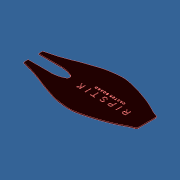
# Autodesk Inventor part: Front Board Cover
Saved by Autodesk Inventor 2018 (Build 220112000, 112)
## iProperties
Created: 2018-03-02
Part Number: Front Board Cover
Material: Generic
Document SubType Name: Modeling
Designer: 232963
Density: 1 g/cm^3
Appearance: Default
Author: 232963
Autodesk Inventor part; units mm, degrees
ref_plane "YZ Plane" through (0, 0, 0) normal (1, 0, 0) x (0, 1, 0)
ref_plane "XZ Plane" through (0, 0, 0) normal (0, 1, 0) x (-1, 0, 0)
ref_plane "XY Plane" through (0, 0, 0) normal (0, 0, 1) x (1, 0, 0)
sketch "Sketch1" plane through (0, 0, 0) normal (0, 0, 1) x (1, 0, 0)
  line L0 (-34.346, 0) -> (308.554, 0)
  line L1 (-34.346, 2.794) -> (-34.346, 0)
  line L2 (-34.346, 2.794) -> (308.554, 2.794)
  line L3 (308.554, 2.794) -> (308.554, 0)
  point P0 (0, 0)
  dimension "d102" = 342.9
  constraints: 8 end point, 1 horizontal, 1 vertical, 1 other
  measures "d102" distance from line of L0.end L1
extrude "Extrusion1" add sketch "Sketch1" along normal blind 161.925
sketch "Sketch2" plane through (-34.346, 2.794, 0) normal (0, 1, 0) x (1, 0, 0)
  line L0 (0, 0) -> (0, -161.925) projected
  line L1 (0, -80.9625) -> (355.6, -80.9625)
  line L2 (342.9, 0) -> (0, 0) projected
  line L3 (0, 0) -> (342.9, 0) projected
  spline S0 degree 4 poles (190.5, 0) (176.6775, 0) (146.1194, -4.9047) (146.8521, -3.1203) (83.6356, -24.6252) (79.4605, -26.74) (68.0118, -31.1235) (63.3839, -33.2828) (38.0924, -42.0424) (22.0487, -47.0453) (18.7736, -46.718) (0.7177, -52.7069) (0, -52.4002) knots 0 0 0 0 0 0.204521 0.323697 0.422378 0.506708 0.581474 0.662125 0.742434 0.828574 1 1 1 1 1
  line L4 (0, -52.4002) -> (0, 0)
  line L5 (190.5, 0) -> (0, 0)
  line L6 (342.9, 0) -> (342.9, -161.925) projected
  spline S1 degree 4 poles (190.5, 0) (208.4411, 0) (251.3479, -12.7353) (261.4383, -16.5213) (279.9875, -22.867) (307.7965, -33.882) (329.1012, -47.2629) (336.8853, -48.836) (342.9, -49.53) knots 0 0 0 0 0 0.297202 0.471636 0.622976 0.773941 1 1 1 1 1
  line L7 (324.9507, -47.459) -> (360.8493, -51.601) construction
  arc A0 (328.7385, -47.0401) -> (357.2564, -50.3305) centre (356.8343, 71.2391) ccw construction
  line L8 (199.9843, 0) -> (190.5, 0)
  point P0 (34.346, 0)
  point P1 (0, -112.0775)
  point P2 (184.15, -161.925)
  point P3 (6.35, -50.8)
  point P4 (19.05, -47.244)
  point P5 (25.4, -45.72)
  point P6 (63.5, -33.02)
  point P7 (38.1, -41.91)
  point P8 (76.2, -27.94)
  point P9 (127, -10.16)
  point P10 (152.4, -3.81)
  point P11 (69.85, -30.48)
  point P12 (82.55, -25.4)
  point P13 (266.7, -18.288)
  point P14 (279.4, -22.86)
  point P15 (304.8, -33.655)
  point P16 (330.2, -46.355)
  point P17 (342.9, -49.53)
  dimension "d8" = 31.115
  dimension "d9" = 184.15
  dimension "d12" = 52.4002
  dimension "d13" = 50.8
  dimension "d15" = 47.244
  dimension "d16" = 6.35
  dimension "d19" = 6.35
  dimension "d20" = 45.72
  dimension "d31" = 41.91
  dimension "d35" = 33.02
  dimension "d37" = 27.94
  dimension "d38" = 12.7
  dimension "d45" = 10.16
  dimension "d49" = 3.81
  dimension "d57" = 30.48
  dimension "d58" = 6.35
  dimension "d60" = 25.4
  dimension "d89" = 190.5
  dimension "d95" = 12.7
  dimension "d96" = 12.7
  dimension "d107" = 13.97
  dimension "d108" = 18.288
  dimension "d109" = 22.86
  dimension "d111" = 33.655
  dimension "d112" = 46.355
  dimension "d113" = 25.4
  dimension "d114" = 49.53
  constraints: 10 end point, 5 point on line, 3 collinear, 3 midpoint, 2 horizontal, 1 centre point, 1 point on circle, 21 other
  measures "d8" distance of point (0, -112.078) L1.start
  measures "d9" distance of L0.end point (184.15, -161.925)
  measures "d12" distance from line of L2 L4.start
  measures "d13" distance from line of L2 point (6.35, -50.8)
  measures "d15" distance from line of L2 point (19.05, -47.244)
  measures "d16" horizontal distance of point (6.35, -50.8) L4.start
  measures "d19" horizontal distance of point (25.4, -45.72) point (19.05, -47.244)
  measures "d20" distance from line of L2 point (25.4, -45.72)
  measures "d31" distance from line of L2 point (38.1, -41.91)
  measures "d35" distance from line of L2 point (63.5, -33.02)
  measures "d37" distance from line of L2 point (76.2, -27.94)
  measures "d38" horizontal distance of point (63.5, -33.02) point (76.2, -27.94)
  measures "d45" distance from line of L2 point (127, -10.16)
  measures "d49" distance from line of L2 point (152.4, -3.81)
  measures "d57" distance from line of L2 point (69.85, -30.48)
  measures "d58" horizontal distance of point (76.2, -27.94) point (69.85, -30.48)
  measures "d60" distance from line of L2 point (82.55, -25.4)
  measures "d89" horizontal distance of L5.start L4.start
  measures "d95" horizontal distance of point (266.7, -18.288) point (254, -13.97)
  measures "d96" horizontal distance of point (279.4, -22.86) point (266.7, -18.288)
  measures "d107" distance from line of L2 point (254, -13.97)
  measures "d108" distance from line of L2 point (266.7, -18.288)
  measures "d109" distance from line of L2 point (279.4, -22.86)
  measures "d111" distance from line of L2 point (304.8, -33.655)
  measures "d112" distance from line of L2 point (330.2, -46.355)
  measures "d113" horizontal distance of point (304.8, -33.655) point (330.2, -46.355)
  measures "d114" distance from line of point (342.9, -49.53) L2
extrude "Extrusion2" cut sketch "Sketch2" against normal blind 25.4 contours L2 S0 L0 | L2 L6 S1
ref_plane "Work Plane2" through (0, 0, 80.9625) normal (0, 0, -1) x (-1, 0, 0)
mirror "Mirror1" about plane through (0, 0, 80.9625) normal (0, 0, -1) of "Extrusion2"
sketch "Sketch3" plane through (308.554, 2.794, 161.925) normal (0, 1, 0) x (1, 0, 0)
  line L0 (-342.9, 109.5248) -> (-342.9, 52.4002) projected
  line L1 (-342.9, 97.6249) -> (-273.05, 97.6249)
  line L2 (-234.95, 96.0374) -> (-234.95, 9.9368) construction
  line L3 (-273.05, 65.8749) -> (-342.9, 65.8749)
  line L4 (-342.9, 65.8749) -> (-342.9, 97.6249)
  line L5 (-273.05, 97.6249) -> (-273.05, 65.8749)
  arc A0 (-273.05, 65.8749) -> (-238.76, 74.1299) centre (-273.05, 141.2201) ccw
  arc A1 (-238.76, 89.3699) -> (-273.05, 97.6249) centre (-273.05, 22.2797) ccw
  line L6 (-238.76, 96.0374) -> (-238.76, 64.2874) construction
  spline S0 degree 4 poles (-238.76, 74.1299) (-236.6016, 75.2331) (-232.3793, 77.6246) (-232.3793, 85.8752) (-236.6016, 88.2667) (-238.76, 89.3699) knots 0 0 0 0 0 0.5 1 1 1 1 1
  point P0 (-308.554, 161.925)
  dimension "d75" = 31.75
  dimension "d78" = 57.1246
  dimension "d79" = 11.8999
  dimension "d80" = 38.1
  dimension "d81" = 15.24
  dimension "d82" = 0
  dimension "d83" = 8.255
  dimension "d84" = 3.81
  dimension "d85" = 0
  dimension "d86" = 107.95
  constraints: 12 end point, 4 point on circle, 2 centre point, 2 parallel, 2 perpendicular, 2 tangent, 1 horizontal, 1 point on line, 1 vertical, 4 other
  measures "d75" distance between parallel lines of L3 L1
  measures "d78" distance of L0.end L0.start
  measures "d79" distance of L0.start L1.start
  measures "d80" distance between parallel lines of L2 L5
  measures "d81" distance of A0.end A1.start
  measures "d82" horizontal distance of A0.end A1.start
  measures "d83" distance from line of A0.end L3
  measures "d84" distance between parallel lines of L6 L2
  measures "d85" distance from line of L6 A1.start
  measures "d86" distance from line of L2 L3.end
extrude "Extrusion3" cut sketch "Sketch3" against normal blind 25.4
fillet "Fillet1" radius 5.715 1 edges at (308.554, 1.397, 49.53)
fillet "Fillet2" radius 5.715 1 edges at (308.554, 1.397, 112.395)
sketch "Sketch4" plane through (-34.346, 2.794, 64.3001) normal (0, 1, 0) x (1, 0, 0)
  line L0 (292.9191, -30.9357) -> (86.9557, -30.9357) construction
  line L1 (86.9557, -30.9357) -> (86.9557, -10.5653) construction
  line L2 (86.9557, -10.5653) -> (292.9191, -10.5653) construction
  line L3 (292.9191, -10.5653) -> (292.9191, -30.9357) construction
  line L4 (261.7969, -5.5259) -> (138.9964, -5.5259) construction
  line L5 (138.9964, -5.5259) -> (138.9964, 7.7104) construction
  line L6 (138.9964, 7.7104) -> (261.7969, 7.7104) construction
  line L7 (261.7969, 7.7104) -> (261.7969, -5.5259) construction
  spline S0 degree 2 poles (279.0348, -25.5302) (279.0348, -22.9286) (280.7333, -21.6346) knots 0 0 0 1 1 1
  spline S1 degree 2 poles (280.7333, -21.6346) (281.9061, -20.7584) (283.0114, -20.7584) knots 0 0 0 1 1 1
  line L8 (283.0114, -20.7584) -> (283.9146, -20.7584)
  line L9 (283.9146, -20.7584) -> (279.1831, -14.0993)
  spline S2 degree 2 poles (279.1831, -14.0993) (279.0348, -13.8701) (279.0348, -13.614) knots 0 0 0 1 1 1
  spline S3 degree 2 poles (279.0348, -13.614) (279.0348, -13.304) (279.5201, -12.8187) (279.8301, -12.8187) knots 0 0 0 1 2 2 2
  spline S4 degree 2 poles (279.8301, -12.8187) (280.2211, -12.8187) (280.4502, -13.1557) knots 0 0 0 1 1 1
  line L10 (280.4502, -13.1557) -> (285.8961, -20.7584)
  line L11 (285.8961, -20.7584) -> (289.9131, -20.7584)
  line L12 (289.9131, -20.7584) -> (289.9131, -13.641)
  spline S5 degree 2 poles (289.9131, -13.641) (289.9131, -12.8187) (290.7084, -12.8187) knots 0 0 0 1 1 1
  spline S6 degree 2 poles (290.7084, -12.8187) (291.5172, -12.8187) (291.5172, -13.641) knots 0 0 0 1 1 1
  line L13 (291.5172, -13.641) -> (291.5172, -30.4909)
  line L14 (291.5172, -30.4909) -> (283.982, -30.4909)
  spline S7 degree 2 poles (283.982, -30.4909) (281.9735, -30.4909) (280.5581, -29.1968) knots 0 0 0 1 1 1
  spline S8 degree 2 poles (280.5581, -29.1968) (279.0348, -27.8084) (279.0348, -25.5302) knots 0 0 0 1 1 1
  spline S9 degree 2 poles (280.612, -25.5302) (280.612, -27.0804) (281.6365, -28.0375) knots 0 0 0 1 1 1
  spline S10 degree 2 poles (281.6365, -28.0375) (282.5935, -28.8867) (283.982, -28.8867) knots 0 0 0 1 1 1
  line L15 (283.982, -28.8867) -> (289.9131, -28.8867)
  line L16 (289.9131, -28.8867) -> (289.9131, -22.3894)
  line L17 (289.9131, -22.3894) -> (283.0114, -22.3894)
  spline S11 degree 2 poles (283.0114, -22.3894) (282.3374, -22.3894) (281.623, -23.0095) knots 0 0 0 1 1 1
  spline S12 degree 2 poles (281.623, -23.0095) (280.612, -23.8587) (280.612, -25.5302) knots 0 0 0 1 1 1
  spline S13 degree 2 poles (263.0881, -13.641) (263.0881, -12.8187) (263.8699, -12.8187) knots 0 0 0 1 1 1
  spline S14 degree 2 poles (263.8699, -12.8187) (264.6653, -12.8187) (264.6653, -13.641) knots 0 0 0 1 1 1
  line L18 (264.6653, -13.641) -> (264.6653, -29.7225)
  spline S15 degree 2 poles (264.6653, -29.7225) (264.6653, -30.5448) (263.8699, -30.5448) knots 0 0 0 1 1 1
  spline S16 degree 2 poles (263.8699, -30.5448) (263.0881, -30.5448) (263.0881, -29.7225) knots 0 0 0 1 1 1
  line L19 (263.0881, -29.7225) -> (263.0881, -13.641)
  spline S17 degree 2 poles (236.6944, -25.9481) (236.6944, -23.9801) (237.7324, -22.8208) knots 0 0 0 1 1 1
  spline S18 degree 2 poles (237.7324, -22.8208) (238.8108, -21.5806) (240.7519, -21.5806) knots 0 0 0 1 1 1
  line L20 (240.7519, -21.5806) -> (246.373, -21.5806)
  line L21 (246.373, -21.5806) -> (246.373, -13.614)
  spline S19 degree 2 poles (246.373, -13.614) (246.373, -12.7917) (247.1548, -12.7917) knots 0 0 0 1 1 1
  spline S20 degree 2 poles (247.1548, -12.7917) (247.9502, -12.7917) (247.9502, -13.614) knots 0 0 0 1 1 1
  line L22 (247.9502, -13.614) -> (247.9502, -30.5178)
  line L23 (247.9502, -30.5178) -> (241.1832, -30.5178)
  spline S21 degree 2 poles (241.1832, -30.5178) (238.9186, -30.5178) (237.7594, -29.2237) knots 0 0 0 1 1 1
  spline S22 degree 2 poles (237.7594, -29.2237) (236.6944, -28.0375) (236.6944, -25.9481) knots 0 0 0 1 1 1
  spline S23 degree 2 poles (238.2716, -25.9481) (238.2716, -28.9137) (241.1832, -28.9137) knots 0 0 0 1 1 1
  line L24 (241.1832, -28.9137) -> (246.373, -28.9137)
  line L25 (246.373, -28.9137) -> (246.373, -23.2117)
  line L26 (246.373, -23.2117) -> (240.7519, -23.2117)
  spline S24 degree 2 poles (240.7519, -23.2117) (239.5657, -23.2117) (238.2716, -24.708) (238.2716, -25.9481) knots 0 0 0 1 2 2 2
  spline S25 degree 2 poles (211.7836, -17.5367) (211.7836, -12.6839) (217.9978, -12.6839) knots 0 0 0 1 1 1
  spline S26 degree 2 poles (217.9978, -12.6839) (221.7452, -12.6839) (223.7807, -16.4043) knots 0 0 0 1 1 1
  spline S27 degree 2 poles (223.7807, -16.4043) (223.8885, -16.6065) (223.8885, -16.8357) knots 0 0 0 1 1 1
  spline S28 degree 2 poles (223.8885, -16.8357) (223.8885, -17.1997) (223.4032, -17.7389) (223.0932, -17.7389) knots 0 0 0 1 2 2 2
  spline S29 degree 2 poles (223.0932, -17.7389) (222.7293, -17.7389) (222.5271, -17.3345) knots 0 0 0 1 1 1
  spline S30 degree 2 poles (222.5271, -17.3345) (221.8531, -15.9056) (219.3728, -14.288) (218.0113, -14.288) knots 0 0 0 1 2 2 2
  spline S31 degree 2 poles (218.0113, -14.288) (213.3877, -14.288) (213.3877, -17.5097) knots 0 0 0 1 1 1
  spline S32 degree 2 poles (213.3877, -17.5097) (213.3877, -18.8577) (214.7222, -19.7608) knots 0 0 0 1 1 1
  spline S33 degree 2 poles (214.7222, -19.7608) (215.6119, -20.3809) (217.7956, -21.1493) knots 0 0 0 1 1 1
  spline S34 degree 2 poles (217.7956, -21.1493) (220.7881, -22.2142) (221.8261, -22.9286) knots 0 0 0 1 1 1
  spline S35 degree 2 poles (221.8261, -22.9286) (223.7537, -24.2497) (223.7537, -26.366) knots 0 0 0 1 1 1
  spline S36 degree 2 poles (223.7537, -26.366) (223.7537, -28.6576) (222.0283, -29.8169) knots 0 0 0 1 1 1
  spline S37 degree 2 poles (222.0283, -29.8169) (220.6399, -30.7739) (218.3618, -30.8548) knots 0 0 0 1 1 1
  spline S38 degree 2 poles (218.3618, -30.8548) (216.2724, -30.9357) (214.7222, -30.0325) knots 0 0 0 1 1 1
  spline S39 degree 2 poles (214.7222, -30.0325) (213.0507, -29.0485) (212.4845, -27.1883) knots 0 0 0 1 1 1
  spline S40 degree 2 poles (212.4845, -27.1883) (212.4306, -27.0535) (212.4306, -26.9322) knots 0 0 0 1 1 1
  spline S41 degree 2 poles (212.4306, -26.9322) (212.4306, -26.2042) (213.2529, -26.2042) knots 0 0 0 1 1 1
  spline S42 degree 2 poles (213.2529, -26.2042) (213.846, -26.2042) (214.0347, -26.7704) knots 0 0 0 1 1 1
  spline S43 degree 2 poles (214.0347, -26.7704) (214.4121, -27.9566) (216.8385, -29.3046) (218.3078, -29.2507) knots 0 0 0 1 2 2 2
  spline S44 degree 2 poles (218.3078, -29.2507) (222.1766, -29.1024) (222.1766, -26.4064) knots 0 0 0 1 1 1
  spline S45 degree 2 poles (222.1766, -26.4064) (222.1766, -24.6271) (219.4941, -23.4948) knots 0 0 0 1 1 1
  spline S46 degree 2 poles (219.4941, -23.4948) (216.9868, -22.5107) (214.4661, -21.5402) knots 0 0 0 1 1 1
  spline S47 degree 2 poles (214.4661, -21.5402) (211.7836, -20.0709) (211.7836, -17.5367) knots 0 0 0 1 1 1
  line L27 (186.5492, -28.8463) -> (191.5233, -28.8463)
  line L28 (191.5233, -28.8463) -> (191.5233, -13.1961)
  spline S48 degree 2 poles (191.5233, -13.1961) (191.5233, -12.3739) (192.3455, -12.3739) knots 0 0 0 1 1 1
  spline S49 degree 2 poles (192.3455, -12.3739) (193.1813, -12.3739) (193.1813, -13.1961) knots 0 0 0 1 1 1
  line L29 (193.1813, -13.1961) -> (193.1813, -28.8463)
  line L30 (193.1813, -28.8463) -> (198.1689, -28.8463)
  spline S50 degree 2 poles (198.1689, -28.8463) (198.9911, -28.8463) (198.9911, -29.6955) knots 0 0 0 1 1 1
  spline S51 degree 2 poles (198.9911, -29.6955) (198.9911, -30.5178) (198.1689, -30.5178) knots 0 0 0 1 1 1
  line L31 (198.1689, -30.5178) -> (186.5492, -30.5178)
  spline S52 degree 2 poles (186.5492, -30.5178) (185.7269, -30.5178) (185.7269, -29.6955) knots 0 0 0 1 1 1
  spline S53 degree 2 poles (185.7269, -29.6955) (185.7269, -28.8463) (186.5492, -28.8463) knots 0 0 0 1 1 1
  spline S54 degree 2 poles (169.7397, -13.641) (169.7397, -12.8187) (170.5216, -12.8187) knots 0 0 0 1 1 1
  spline S55 degree 2 poles (170.5216, -12.8187) (171.3169, -12.8187) (171.3169, -13.641) knots 0 0 0 1 1 1
  line L32 (171.3169, -13.641) -> (171.3169, -29.7225)
  spline S56 degree 2 poles (171.3169, -29.7225) (171.3169, -30.5448) (170.5216, -30.5448) knots 0 0 0 1 1 1
  spline S57 degree 2 poles (170.5216, -30.5448) (169.7397, -30.5448) (169.7397, -29.7225) knots 0 0 0 1 1 1
  line L33 (169.7397, -29.7225) -> (169.7397, -13.641)
  spline S58 degree 2 poles (142.8878, -14.0319) (142.7664, -13.8162) (142.7664, -13.614) knots 0 0 0 1 1 1
  spline S59 degree 2 poles (142.7664, -13.614) (142.7664, -13.277) (143.2787, -12.8187) (143.6157, -12.8187) knots 0 0 0 1 2 2 2
  spline S60 degree 2 poles (143.6157, -12.8187) (144.0066, -12.8187) (144.2357, -13.1961) knots 0 0 0 1 1 1
  line L34 (144.2357, -13.1961) -> (150.3152, -23.6431)
  line L35 (150.3152, -23.6431) -> (153.0516, -21.0414)
  line L36 (153.0516, -21.0414) -> (153.0516, -13.641)
  spline S61 degree 2 poles (153.0516, -13.641) (153.0516, -12.8187) (153.8334, -12.8187) knots 0 0 0 1 1 1
  spline S62 degree 2 poles (153.8334, -12.8187) (154.6288, -12.8187) (154.6288, -13.641) knots 0 0 0 1 1 1
  line L37 (154.6288, -13.641) -> (154.6288, -29.6955)
  spline S63 degree 2 poles (154.6288, -29.6955) (154.6288, -30.5178) (153.8334, -30.5178) knots 0 0 0 1 1 1
  spline S64 degree 2 poles (153.8334, -30.5178) (153.0516, -30.5178) (153.0516, -29.6955) knots 0 0 0 1 1 1
  line L38 (153.0516, -29.6955) -> (153.0516, -23.2117)
  line L39 (153.0516, -23.2117) -> (145.4489, -30.2617)
  spline S65 degree 2 poles (145.4489, -30.2617) (145.2063, -30.5178) (144.8963, -30.5178) knots 0 0 0 1 1 1
  spline S66 degree 2 poles (144.8963, -30.5178) (144.5862, -30.5178) (144.1279, -30.0191) (144.1279, -29.6955) knots 0 0 0 1 2 2 2
  spline S67 degree 2 poles (144.1279, -29.6955) (144.1279, -29.3585) (144.411, -29.1024) knots 0 0 0 1 1 1
  line L40 (144.411, -29.1024) -> (149.1559, -24.7349)
  line L41 (149.1559, -24.7349) -> (142.8878, -14.0319)
  spline S68 degree 2 poles (258.6733, 1.0711) (259.2908, 1.0711) (260.3355, 0.6543) (260.7163, 0.2375) knots 0 0 0 1 2 2 2
  spline S69 degree 2 poles (260.7163, 0.2375) (261.097, -0.1742) (261.5139, -1.4092) (261.5139, -2.2119) knots 0 0 0 1 2 2 2
  spline S70 degree 2 poles (261.5139, -2.2119) (261.5139, -3.0095) (261.1073, -4.1931) (260.7214, -4.6305) knots 0 0 0 1 2 2 2
  spline S71 degree 2 poles (260.7214, -4.6305) (260.3406, -5.0576) (259.3011, -5.5053) (258.6579, -5.5053) knots 0 0 0 1 2 2 2
  spline S72 degree 2 poles (258.6579, -5.5053) (258.3389, -5.5053) (257.778, -5.4127) (257.5413, -5.3406) knots 0 0 0 1 2 2 2
  spline S73 degree 2 poles (257.5413, -5.3406) (257.3354, -5.2737) (256.9083, -5.0833) (256.6973, -4.9701) knots 0 0 0 1 2 2 2
  line L42 (256.6973, -4.9701) -> (256.6973, -3.9512)
  line L43 (256.6973, -3.9512) -> (256.7642, -3.9512)
  spline S74 degree 2 poles (256.7642, -3.9512) (256.8774, -4.0542) (257.2274, -4.3423) (257.4795, -4.4813) knots 0 0 0 1 2 2 2
  spline S75 degree 2 poles (257.4795, -4.4813) (257.7214, -4.6151) (258.2925, -4.7849) (258.6631, -4.7849) knots 0 0 0 1 2 2 2
  spline S76 degree 2 poles (258.6631, -4.7849) (259.0696, -4.7849) (259.7951, -4.4504) (260.0679, -4.1313) knots 0 0 0 1 2 2 2
  spline S77 degree 2 poles (260.0679, -4.1313) (260.3355, -3.8072) (260.6339, -2.8243) (260.6339, -2.2119) knots 0 0 0 1 2 2 2
  spline S78 degree 2 poles (260.6339, -2.2119) (260.6339, -1.5584) (260.32, -0.6167) (260.0473, -0.2925) knots 0 0 0 1 2 2 2
  spline S79 degree 2 poles (260.0473, -0.2925) (259.7797, 0.0214) (259.0644, 0.3404) (258.6631, 0.3404) knots 0 0 0 1 2 2 2
  spline S80 degree 2 poles (258.6631, 0.3404) (258.2977, 0.3404) (257.675, 0.1603) (257.4332, 0.0265) knots 0 0 0 1 2 2 2
  spline S81 degree 2 poles (257.4332, 0.0265) (257.2016, -0.1073) (256.8569, -0.3852) (256.7591, -0.4829) knots 0 0 0 1 2 2 2
  line L44 (256.7591, -0.4829) -> (256.6973, -0.4829)
  line L45 (256.6973, -0.4829) -> (256.6973, 0.5257)
  spline S82 degree 2 poles (256.6973, 0.5257) (256.9083, 0.6234) (257.2788, 0.8035) (257.5413, 0.8859) knots 0 0 0 1 2 2 2
  spline S83 degree 2 poles (257.5413, 0.8859) (257.8191, 0.9785) (258.2925, 1.0711) (258.6733, 1.0711) knots 0 0 0 1 2 2 2
  line L46 (253.8671, 0.9579) -> (251.7264, -5.3921)
  line L47 (251.7264, -5.3921) -> (250.687, -5.3921)
  line L48 (250.687, -5.3921) -> (248.5463, 0.9579)
  line L49 (248.5463, 0.9579) -> (249.4365, 0.9579)
  line L50 (249.4365, 0.9579) -> (250.0128, -0.8174)
  line L51 (250.0128, -0.8174) -> (252.4366, -0.8174)
  line L52 (252.4366, -0.8174) -> (253.0129, 0.9579)
  line L53 (253.0129, 0.9579) -> (253.8671, 0.9579)
  line L54 (250.2444, -1.5378) -> (251.2273, -4.5276)
  line L55 (251.2273, -4.5276) -> (252.205, -1.5378)
  line L56 (252.205, -1.5378) -> (250.2444, -1.5378)
  spline S84 degree 2 poles (243.4467, 1.0711) (244.1363, 1.0711) (245.1037, 0.783) (245.5308, 0.5771) knots 0 0 0 1 2 2 2
  line L57 (245.5308, 0.5771) -> (245.5308, -0.4829)
  line L58 (245.5308, -0.4829) -> (245.469, -0.4829)
  spline S85 degree 2 poles (245.469, -0.4829) (245.0522, -0.0918) (243.9973, 0.3404) (243.5085, 0.3404) knots 0 0 0 1 2 2 2
  spline S86 degree 2 poles (243.5085, 0.3404) (242.8086, 0.3404) (242.0934, -0.2411) (242.0934, -0.7196) knots 0 0 0 1 2 2 2
  spline S87 degree 2 poles (242.0934, -0.7196) (242.0934, -1.1004) (242.469, -1.5738) (242.8755, -1.6922) knots 0 0 0 1 2 2 2
  spline S88 degree 2 poles (242.8755, -1.6922) (243.1688, -1.7745) (243.6577, -1.8877) (244.0231, -1.9804) knots 0 0 0 1 2 2 2
  spline S89 degree 2 poles (244.0231, -1.9804) (244.3524, -2.0679) (244.8721, -2.3303) (245.0728, -2.5413) knots 0 0 0 1 2 2 2
  spline S90 degree 2 poles (245.0728, -2.5413) (245.2684, -2.7523) (245.4845, -3.3183) (245.4845, -3.6888) knots 0 0 0 1 2 2 2
  spline S91 degree 2 poles (245.4845, -3.6888) (245.4845, -4.4607) (244.2804, -5.5053) (243.3489, -5.5053) knots 0 0 0 1 2 2 2
  spline S92 degree 2 poles (243.3489, -5.5053) (242.8138, -5.5053) (241.8669, -5.2943) (241.4604, -5.0936) knots 0 0 0 1 2 2 2
  line L59 (241.4604, -5.0936) -> (241.4604, -4.085)
  line L60 (241.4604, -4.085) -> (241.5222, -4.085)
  spline S93 degree 2 poles (241.5222, -4.085) (241.8258, -4.3629) (242.7726, -4.7746) (243.2923, -4.7746) knots 0 0 0 1 2 2 2
  spline S94 degree 2 poles (243.2923, -4.7746) (243.879, -4.7746) (244.6045, -4.224) (244.6045, -3.7763) knots 0 0 0 1 2 2 2
  spline S95 degree 2 poles (244.6045, -3.7763) (244.6045, -3.3749) (244.1774, -2.8963) (243.7761, -2.7883) knots 0 0 0 1 2 2 2
  spline S96 degree 2 poles (243.7761, -2.7883) (243.5085, -2.7162) (242.7314, -2.531) (242.4742, -2.4538) knots 0 0 0 1 2 2 2
  spline S97 degree 2 poles (242.4742, -2.4538) (241.8206, -2.2531) (241.2134, -1.4452) (241.2134, -0.8534) knots 0 0 0 1 2 2 2
  spline S98 degree 2 poles (241.2134, -0.8534) (241.2134, -0.4778) (241.517, 0.2426) (241.7898, 0.4948) knots 0 0 0 1 2 2 2
  spline S99 degree 2 poles (241.7898, 0.4948) (242.0934, 0.7727) (242.8652, 1.0711) (243.4467, 1.0711) knots 0 0 0 1 2 2 2
  line L61 (236.1447, 0.9579) -> (236.1447, -4.6408)
  line L62 (236.1447, -4.6408) -> (238.2751, -4.6408)
  line L63 (238.2751, -4.6408) -> (238.2751, -5.3921)
  line L64 (238.2751, -5.3921) -> (233.1704, -5.3921)
  line L65 (233.1704, -5.3921) -> (233.1704, -4.6408)
  line L66 (233.1704, -4.6408) -> (235.3008, -4.6408)
  line L67 (235.3008, -4.6408) -> (235.3008, 0.9579)
  line L68 (235.3008, 0.9579) -> (236.1447, 0.9579)
  line L69 (229.7999, 0.9579) -> (229.7999, -5.3921)
  line L70 (229.7999, -5.3921) -> (225.8273, -5.3921)
  line L71 (225.8273, -5.3921) -> (225.8273, -4.6408)
  line L72 (225.8273, -4.6408) -> (228.956, -4.6408)
  line L73 (228.956, -4.6408) -> (228.956, -2.9015)
  line L74 (228.956, -2.9015) -> (226.0383, -2.9015)
  line L75 (226.0383, -2.9015) -> (226.0383, -2.1502)
  line L76 (226.0383, -2.1502) -> (228.956, -2.1502)
  line L77 (228.956, -2.1502) -> (228.956, 0.2066)
  line L78 (228.956, 0.2066) -> (225.8273, 0.2066)
  line L79 (225.8273, 0.2066) -> (225.8273, 0.9579)
  line L80 (225.8273, 0.9579) -> (229.7999, 0.9579)
  line L81 (217.2594, 0.9579) -> (218.3555, 0.9579)
  line L82 (218.3555, 0.9579) -> (220.3624, -1.5687)
  line L83 (220.3624, -1.5687) -> (221.3298, -1.5687)
  line L84 (221.3298, -1.5687) -> (221.3298, 0.9579)
  line L85 (221.3298, 0.9579) -> (222.1737, 0.9579)
  line L86 (222.1737, 0.9579) -> (222.1737, -5.3921)
  line L87 (222.1737, -5.3921) -> (220.5373, -5.3921)
  spline S100 degree 2 poles (220.5373, -5.3921) (219.9919, -5.3921) (219.256, -5.2737) (218.9215, -5.0576) knots 0 0 0 1 2 2 2
  spline S101 degree 2 poles (218.9215, -5.0576) (218.587, -4.8415) (218.2011, -4.1674) (218.2011, -3.6682) knots 0 0 0 1 2 2 2
  spline S102 degree 2 poles (218.2011, -3.6682) (218.2011, -2.9735) (218.9112, -2.0318) (219.5184, -1.8054) knots 0 0 0 1 2 2 2
  line L88 (219.5184, -1.8054) -> (217.2594, 0.9579)
  spline S103 degree 2 poles (219.081, -3.6013) (219.081, -3.8792) (219.2766, -4.3063) (219.4824, -4.4452) knots 0 0 0 1 2 2 2
  spline S104 degree 2 poles (219.4824, -4.4452) (219.6625, -4.5636) (220.1411, -4.6614) (220.491, -4.6614) knots 0 0 0 1 2 2 2
  line L89 (220.491, -4.6614) -> (221.3298, -4.6614)
  line L90 (221.3298, -4.6614) -> (221.3298, -2.2737)
  line L91 (221.3298, -2.2737) -> (220.5888, -2.2737)
  spline S105 degree 2 poles (220.5888, -2.2737) (220.2234, -2.2737) (219.6419, -2.4023) (219.4413, -2.603) knots 0 0 0 1 2 2 2
  spline S106 degree 2 poles (219.4413, -2.603) (219.256, -2.778) (219.081, -3.272) (219.081, -3.6013) knots 0 0 0 1 2 2 2
  spline S107 degree 2 poles (206.9934, -0.9924) (206.9934, -0.5189) (207.3536, 0.2066) (207.6521, 0.4433) knots 0 0 0 1 2 2 2
  spline S108 degree 2 poles (207.6521, 0.4433) (208.0123, 0.7212) (208.8305, 0.9579) (209.4789, 0.9579) knots 0 0 0 1 2 2 2
  line L92 (209.4789, 0.9579) -> (211.3005, 0.9579)
  line L93 (211.3005, 0.9579) -> (211.3005, -5.3921)
  line L94 (211.3005, -5.3921) -> (209.6178, -5.3921)
  spline S109 degree 2 poles (209.6178, -5.3921) (208.9385, -5.3921) (208.2593, -5.3046) (207.9505, -5.1348) knots 0 0 0 1 2 2 2
  spline S110 degree 2 poles (207.9505, -5.1348) (207.6058, -4.9547) (207.2919, -4.3629) (207.2919, -3.9615) knots 0 0 0 1 2 2 2
  spline S111 degree 2 poles (207.2919, -3.9615) (207.2919, -3.5138) (207.7653, -2.8037) (208.1821, -2.603) knots 0 0 0 1 2 2 2
  line L95 (208.1821, -2.603) -> (208.1821, -2.5721)
  spline S112 degree 2 poles (208.1821, -2.5721) (207.616, -2.4178) (206.9934, -1.5996) (206.9934, -0.9924) knots 0 0 0 1 2 2 2
  spline S113 degree 2 poles (207.8733, -0.9563) (207.8733, -1.3166) (208.0792, -1.7797) (208.3879, -1.9444) knots 0 0 0 1 2 2 2
  spline S114 degree 2 poles (208.3879, -1.9444) (208.5886, -2.0473) (209.062, -2.109) (209.4994, -2.109) knots 0 0 0 1 2 2 2
  line L96 (209.4994, -2.109) -> (210.4566, -2.109)
  line L97 (210.4566, -2.109) -> (210.4566, 0.2375)
  line L98 (210.4566, 0.2375) -> (209.7722, 0.2375)
  spline S115 degree 2 poles (209.7722, 0.2375) (209.2164, 0.2375) (208.5783, 0.1346) (208.3313, -0.0301) knots 0 0 0 1 2 2 2
  spline S116 degree 2 poles (208.3313, -0.0301) (208.0946, -0.1999) (207.8733, -0.6219) (207.8733, -0.9563) knots 0 0 0 1 2 2 2
  spline S117 degree 2 poles (208.1718, -3.8432) (208.1718, -4.0696) (208.3262, -4.4092) (208.496, -4.507) knots 0 0 0 1 2 2 2
  spline S118 degree 2 poles (208.496, -4.507) (208.7018, -4.6202) (209.201, -4.6717) (209.6487, -4.6717) knots 0 0 0 1 2 2 2
  line L99 (209.6487, -4.6717) -> (210.4566, -4.6717)
  line L100 (210.4566, -4.6717) -> (210.4566, -2.814)
  line L101 (210.4566, -2.814) -> (209.4994, -2.814)
  spline S119 degree 2 poles (209.4994, -2.814) (209.1032, -2.814) (208.7276, -2.8963) (208.5269, -3.025) knots 0 0 0 1 2 2 2
  spline S120 degree 2 poles (208.5269, -3.025) (208.3313, -3.1485) (208.1718, -3.5447) (208.1718, -3.8432) knots 0 0 0 1 2 2 2
  spline S121 degree 2 poles (198.935, -4.6665) (198.5748, -4.2446) (198.1734, -3.0095) (198.1734, -2.2171) knots 0 0 0 1 2 2 2
  spline S122 degree 2 poles (198.1734, -2.2171) (198.1734, -1.4452) (198.5645, -0.1948) (198.935, 0.2272) knots 0 0 0 1 2 2 2
  spline S123 degree 2 poles (198.935, 0.2272) (199.3261, 0.6697) (200.3604, 1.0917) (200.983, 1.0917) knots 0 0 0 1 2 2 2
  spline S124 degree 2 poles (200.983, 1.0917) (201.6263, 1.0917) (202.6554, 0.6543) (203.0311, 0.2272) knots 0 0 0 1 2 2 2
  spline S125 degree 2 poles (203.0311, 0.2272) (203.3964, -0.1948) (203.7875, -1.4349) (203.7875, -2.2171) knots 0 0 0 1 2 2 2
  spline S126 degree 2 poles (203.7875, -2.2171) (203.7875, -3.0147) (203.3913, -4.2291) (203.0259, -4.6665) knots 0 0 0 1 2 2 2
  spline S127 degree 2 poles (203.0259, -4.6665) (202.6554, -5.0885) (201.6211, -5.5259) (200.983, -5.5259) knots 0 0 0 1 2 2 2
  spline S128 degree 2 poles (200.983, -5.5259) (200.3346, -5.5259) (199.2952, -5.073) (198.935, -4.6665) knots 0 0 0 1 2 2 2
  spline S129 degree 2 poles (199.0533, -2.2171) (199.0533, -2.8449) (199.3261, -3.8174) (199.5731, -4.1365) knots 0 0 0 1 2 2 2
  spline S130 degree 2 poles (199.5731, -4.1365) (199.8252, -4.4658) (200.5353, -4.7952) (200.9779, -4.7952) knots 0 0 0 1 2 2 2
  spline S131 degree 2 poles (200.9779, -4.7952) (201.4359, -4.7952) (202.1254, -4.4761) (202.3878, -4.1365) knots 0 0 0 1 2 2 2
  spline S132 degree 2 poles (202.3878, -4.1365) (202.64, -3.8123) (202.9076, -2.8346) (202.9076, -2.2171) knots 0 0 0 1 2 2 2
  spline S133 degree 2 poles (202.9076, -2.2171) (202.9076, -0.9666) (201.8578, 0.361) (200.9779, 0.361) knots 0 0 0 1 2 2 2
  spline S134 degree 2 poles (200.9779, 0.361) (200.0979, 0.361) (199.0533, -0.9666) (199.0533, -2.2171) knots 0 0 0 1 2 2 2
  line L102 (195.2042, 0.9579) -> (193.0635, -5.3921)
  line L103 (193.0635, -5.3921) -> (192.0241, -5.3921)
  line L104 (192.0241, -5.3921) -> (189.8834, 0.9579)
  line L105 (189.8834, 0.9579) -> (190.7736, 0.9579)
  line L106 (190.7736, 0.9579) -> (191.35, -0.8174)
  line L107 (191.35, -0.8174) -> (193.7737, -0.8174)
  line L108 (193.7737, -0.8174) -> (194.35, 0.9579)
  line L109 (194.35, 0.9579) -> (195.2042, 0.9579)
  line L110 (191.5815, -1.5378) -> (192.5644, -4.5276)
  line L111 (192.5644, -4.5276) -> (193.5421, -1.5378)
  line L112 (193.5421, -1.5378) -> (191.5815, -1.5378)
  line L113 (181.6397, 0.9579) -> (182.7358, 0.9579)
  line L114 (182.7358, 0.9579) -> (184.7427, -1.5687)
  line L115 (184.7427, -1.5687) -> (185.7101, -1.5687)
  line L116 (185.7101, -1.5687) -> (185.7101, 0.9579)
  line L117 (185.7101, 0.9579) -> (186.554, 0.9579)
  line L118 (186.554, 0.9579) -> (186.554, -5.3921)
  line L119 (186.554, -5.3921) -> (184.9176, -5.3921)
  spline S135 degree 2 poles (184.9176, -5.3921) (184.3722, -5.3921) (183.6363, -5.2737) (183.3018, -5.0576) knots 0 0 0 1 2 2 2
  spline S136 degree 2 poles (183.3018, -5.0576) (182.9673, -4.8415) (182.5814, -4.1674) (182.5814, -3.6682) knots 0 0 0 1 2 2 2
  spline S137 degree 2 poles (182.5814, -3.6682) (182.5814, -2.9735) (183.2915, -2.0318) (183.8987, -1.8054) knots 0 0 0 1 2 2 2
  line L120 (183.8987, -1.8054) -> (181.6397, 0.9579)
  spline S138 degree 2 poles (183.4613, -3.6013) (183.4613, -3.8792) (183.6569, -4.3063) (183.8627, -4.4452) knots 0 0 0 1 2 2 2
  spline S139 degree 2 poles (183.8627, -4.4452) (184.0428, -4.5636) (184.5214, -4.6614) (184.8713, -4.6614) knots 0 0 0 1 2 2 2
  line L121 (184.8713, -4.6614) -> (185.7101, -4.6614)
  line L122 (185.7101, -4.6614) -> (185.7101, -2.2737)
  line L123 (185.7101, -2.2737) -> (184.9691, -2.2737)
  spline S140 degree 2 poles (184.9691, -2.2737) (184.6037, -2.2737) (184.0222, -2.4023) (183.8216, -2.603) knots 0 0 0 1 2 2 2
  spline S141 degree 2 poles (183.8216, -2.603) (183.6363, -2.778) (183.4613, -3.272) (183.4613, -3.6013) knots 0 0 0 1 2 2 2
  spline S142 degree 2 poles (173.4012, -2.2119) (173.4012, -1.3423) (174.1062, 0.0574) (174.6979, 0.4485) knots 0 0 0 1 2 2 2
  spline S143 degree 2 poles (174.6979, 0.4485) (175.1816, 0.7521) (176.1748, 0.9579) (176.9467, 0.9579) knots 0 0 0 1 2 2 2
  line L124 (176.9467, 0.9579) -> (178.4081, 0.9579)
  line L125 (178.4081, 0.9579) -> (178.4081, -5.3921)
  line L126 (178.4081, -5.3921) -> (176.9621, -5.3921)
  spline S144 degree 2 poles (176.9621, -5.3921) (176.0667, -5.3921) (175.0479, -5.1245) (174.6876, -4.8878) knots 0 0 0 1 2 2 2
  spline S145 degree 2 poles (174.6876, -4.8878) (174.0753, -4.4813) (173.4012, -3.1382) (173.4012, -2.2119) knots 0 0 0 1 2 2 2
  spline S146 degree 2 poles (174.2811, -2.2222) (174.2811, -2.9529) (174.7648, -3.9873) (175.2434, -4.2806) knots 0 0 0 1 2 2 2
  spline S147 degree 2 poles (175.2434, -4.2806) (175.583, -4.4813) (176.3498, -4.6614) (176.921, -4.6614) knots 0 0 0 1 2 2 2
  line L127 (176.921, -4.6614) -> (177.5642, -4.6614)
  line L128 (177.5642, -4.6614) -> (177.5642, 0.2272)
  line L129 (177.5642, 0.2272) -> (176.921, 0.2272)
  spline S148 degree 2 poles (176.921, 0.2272) (176.3601, 0.2272) (175.511, 0.0471) (175.1662, -0.1948) knots 0 0 0 1 2 2 2
  spline S149 degree 2 poles (175.1662, -0.1948) (174.7237, -0.4932) (174.2811, -1.4812) (174.2811, -2.2222) knots 0 0 0 1 2 2 2
  point P0 (0, 0)
  constraints: 4 other
extrude "Extrusion4" add sketch "Sketch4" along normal blind 0.254
equation "\"d8\" = d7"
equation "\"d7\" = 31.115"
body "Solid1"
